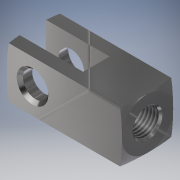
# Autodesk Inventor part: D-14053
Saved by Autodesk Inventor 2017 (Build 210142000, 142)
## iProperties
Category: PARTsolutions
Company: BIMBA
Created: 2016-10-01
Part Number: D-14053
Catalog Web Link: www.cadenas.de
Description: Piston Rod Clevis for Original Line Cylinders - Body-
Vendor: BIMBA
Document SubType Name: Modeling
Designer: psAdmin
Manufacturer: BIMBA
Mass: 70.1826 g
Surface Area: 47.8008 cm^2
Volume: 8.94045 cm^3
Density: 7.85 g/cm^3
Material: Steel, Galvanized
Appearance: Galvanized
PSOL_IDENT_0: {$CADENAS_DATA\23d-libs\bimba\bimba\bimba_imperial\bimba_full_line\original_line_cylinders\accessori
PSOL_IDENT_1: es\piston_rod_clevis_body.prj},202 {VTYP=3D},{NB=D-14053},{LINA=D-14053},{NN=Piston Rod Clevis for O
PSOL_IDENT_2: riginal Line Cylinders - Body},{DATE=22.09.2016 13:52:23},{GEOMDATE=06.12.2012 07:16:06},{VERSION=},
PSOL_IDENT_3: {LINEID=40},{LINESUBID=-1},{WBVAR=}  {NB=D-14053},{LINA=D-14053},{KT=DUMMY},{PN=D-14053},{L=1.688000
PSOL_IDENT_4: 00},{L1=1.31200000},{L2=0.75000000},{W=0.38750000},{W1=0.75000000},{DIA1=0.37200000},{DIA1CS=0.04500
PSOL_IDENT_5: 000},{DIA2=0.75000000},{DIA3=0.39060000},{CS=90.00000000},{CDP=0.03000000},{AN=30.00000000},{NDM=0.4
PSOL_IDENT_6: 3750000},{CODE=UNF},{NDMDP=0.62000000},{COLOR=0.75,0.75,0.75,0.00}
NN: Piston Rod Clevis for Original Line Cylinders - Body
NB: D-14053
NBSYN: $PN.
LINA: D-14053
PN: D-14053
L: 1.68800000
L1: 1.31200000
L2: 0.75000000
W: 0.38750000
W1: 0.75000000
DIA1: 0.37200000
DIA1CS: 0.04500000
DIA2: 0.75000000
DIA3: 0.39060000
CS: 90.00000000
CDP: 0.03000000
AN: 30.00000000
NDM: 0.43750000
CODE: UNF
NDMDP: 0.62000000
SUPPLIER: BIMBA
ARTICLENO: D-14053
BOMINFO: D-14053
CREATOR: CADENAS GmbH
Title: D-14053
Author: Cadenas PARTsolutions
Autodesk Inventor part; units mm, degrees
sketch "Sketch_1" plane through (0, 0, 0) normal (0, 0, 1) x (1, 0, 0)
  line L0 (-9.5504, -9.525) -> (33.3248, -9.525)
  line L1 (33.3248, -9.525) -> (33.3248, 9.525)
  line L2 (33.3248, 9.525) -> (-9.5504, 9.525)
  line L3 (-9.5504, 9.525) -> (-9.5504, -9.525)
  constraints: 8 end point
extrude "Extrusion1" add sketch "Sketch_1" along normal mid plane 19.05
sketch "Sketch_2" plane through (0, 0, 0) normal (0, 1, 0) x (-1, 0, 0)
  line L0 (9.5504, 4.9212) -> (-14.2748, 4.9212)
  line L1 (-14.2748, 4.9212) -> (-14.2748, -4.9212)
  line L2 (-14.2748, -4.9212) -> (9.5504, -4.9212)
  line L3 (9.5504, -4.9212) -> (9.5504, 4.9212)
  constraints: 8 end point
extrude "Extrusion2" cut sketch "Sketch_2" along normal mid plane 19.05
sketch "Sketch_3" plane through (0, 0, 0) normal (0, 0, 1) x (1, 0, 0)
  line L0 (33.3248, 0) -> (17.5768, 0)
  line L1 (17.5768, 0) -> (17.5768, 4.8692)
  line L2 (17.5768, 4.8692) -> (32.6377, 4.8692)
  line L3 (32.6377, 4.8692) -> (33.3248, 5.5563)
  line L4 (33.3248, 5.5563) -> (33.3248, 0)
  line L5 (33.3248, 0) -> (17.5768, 0)
  constraints: 12 end point
revolve "Revolution1" cut sketch "Sketch_3" angle 360 about axis through (33.3248, 0, 0) along (1, 0, 0)
thread "Thread1" size "7/16-20 UNF" class "2B" standard "ANSI Unified Screw Threads" full length
sketch "Sketch5" plane through (17.5768, 0, 0) normal (1, 0, 0) x (0, 0, -1)
  point P0 (0, 0)
hole "Hole1" at (17.5768, 0, 0) direction (-1, 0, 0) diameter 9.9212 depth 3.302
sketch "Sketch_5" plane through (0, 0, 0) normal (1, 0, 0) x (0, 1, 0)
  line L0 (0, -9.525) -> (0, 9.525)
  line L1 (0, 9.525) -> (5.8674, 9.525)
  line L2 (5.8674, 9.525) -> (4.7244, 8.382)
  line L3 (4.7244, 8.382) -> (4.7244, -8.382)
  line L4 (4.7244, -8.382) -> (5.8674, -9.525)
  line L5 (5.8674, -9.525) -> (0, -9.525)
  line L6 (0, -9.525) -> (0, 9.525)
  constraints: 14 end point
revolve "Revolution2" cut sketch "Sketch_5" angle 360 about axis through (0, 0, -9.525) along (0, 0, -1)
sketch "Sketch_9" plane through (0, 0, 0) normal (0, 0, 1) x (1, 0, 0)
  line L0 (42.8498, 0) -> (33.3248, 0)
  line L1 (33.3248, 0) -> (33.3248, 9.525)
  arc A0 (33.3248, 9.525) -> (30.7848, 19.05) centre (-3.664, 4.7625) ccw
  line L2 (30.7848, 19.05) -> (42.8498, 19.05)
  line L3 (42.8498, 19.05) -> (42.8498, 0)
  line L4 (42.8498, 0) -> (33.3248, 0)
  constraints: 10 end point, 2 point on circle, 1 centre point
revolve "Revolution3" cut sketch "Sketch_9" angle 360 about axis through (42.8498, 0, 0) along (1, 0, 0)
sketch "Sketch_10" plane through (0, 0, 0) normal (0, 0, 1) x (1, 0, 0)
  line L0 (-9.5504, 0) -> (-19.0754, 0)
  line L1 (-19.0754, 0) -> (-19.0754, 19.05)
  line L2 (-19.0754, 19.05) -> (-7.0104, 19.05)
  arc A0 (-7.0104, 19.05) -> (-9.5504, 9.525) centre (27.4383, 4.7625) ccw
  line L3 (-9.5504, 9.525) -> (-9.5504, 0)
  line L4 (-9.5504, 0) -> (-19.0754, 0)
  constraints: 10 end point, 2 point on circle, 1 centre point
revolve "Revolution4" cut sketch "Sketch_10" angle 360 about axis through (-9.5504, 0, 0) along (1, 0, 0)
ref_plane "dummy_XY" through (0, 0, 0) normal (0, 0, 1) x (1, 0, 0)
ref_plane "dummy_YZ" through (0, 0, 0) normal (1, 0, 0) x (0, 1, 0)
ref_plane "dummy_ZX" through (0, 0, 0) normal (0, 1, 0) x (0, 0, 1)
ref_plane "h1_XY" through (-9.5504, 9.525, 0) normal (0, 0, 1) x (1, 0, 0)
ref_plane "h1_YZ" through (-9.5504, 9.525, 0) normal (1, 0, 0) x (0, 1, 0)
ref_plane "h1_ZX" through (-9.5504, 9.525, 0) normal (0, 1, 0) x (0, 0, 1)
ref_plane "h2_XY" through (-9.5504, -9.525, 0) normal (0, 0, 1) x (1, 0, 0)
ref_plane "h2_YZ" through (-9.5504, -9.525, 0) normal (1, 0, 0) x (0, 1, 0)
ref_plane "h2_ZX" through (-9.5504, -9.525, 0) normal (0, 1, 0) x (0, 0, 1)
ref_plane "l1_XY" through (33.3248, 9.525, 0) normal (0, 0, 1) x (1, 0, 0)
ref_plane "l1_YZ" through (33.3248, 9.525, 0) normal (1, 0, 0) x (0, 1, 0)
ref_plane "l1_ZX" through (33.3248, 9.525, 0) normal (0, 1, 0) x (0, 0, 1)
ref_plane "l11_XY" through (33.3248, 9.525, 0) normal (0, 0, 1) x (1, 0, 0)
ref_plane "l11_YZ" through (33.3248, 9.525, 0) normal (1, 0, 0) x (0, 1, 0)
ref_plane "l11_ZX" through (33.3248, 9.525, 0) normal (0, 1, 0) x (0, 0, 1)
ref_plane "l12_XY" through (0, 9.525, 0) normal (0, 0, 1) x (1, 0, 0)
ref_plane "l12_YZ" through (0, 9.525, 0) normal (1, 0, 0) x (0, 1, 0)
ref_plane "l12_ZX" through (0, 9.525, 0) normal (0, 1, 0) x (0, 0, 1)
ref_plane "l2_XY" through (-9.5504, 9.525, 0) normal (0, 0, 1) x (1, 0, 0)
ref_plane "l2_YZ" through (-9.5504, 9.525, 0) normal (1, 0, 0) x (0, 1, 0)
ref_plane "l2_ZX" through (-9.5504, 9.525, 0) normal (0, 1, 0) x (0, 0, 1)
ref_plane "l21_XY" through (33.3248, 0, 0) normal (0, 1, 0) x (1, 0, 0)
ref_plane "l21_YZ" through (33.3248, 0, 0) normal (1, 0, 0) x (0, 0, -1)
ref_plane "l21_ZX" through (33.3248, 0, 0) normal (0, 0, -1) x (0, 1, 0)
ref_plane "l22_XY" through (14.2748, 0, 0) normal (0, 1, 0) x (1, 0, 0)
ref_plane "l22_YZ" through (14.2748, 0, 0) normal (1, 0, 0) x (0, 0, -1)
ref_plane "l22_ZX" through (14.2748, 0, 0) normal (0, 0, -1) x (0, 1, 0)
ref_plane "piston_rod_clevis_XY" through (33.3248, 0, 0) normal (1, 0, 0) x (0, 0, -1)
ref_plane "piston_rod_clevis_YZ" through (33.3248, 0, 0) normal (0, 0, -1) x (0, 1, 0)
ref_plane "piston_rod_clevis_ZX" through (33.3248, 0, 0) normal (0, 1, 0) x (1, 0, 0)
ref_plane "rod_clevis_body_XY" through (0, 0, 0) normal (0, 0, 1) x (1, 0, 0)
ref_plane "rod_clevis_body_YZ" through (0, 0, 0) normal (1, 0, 0) x (0, 1, 0)
ref_plane "rod_clevis_body_ZX" through (0, 0, 0) normal (0, 1, 0) x (0, 0, 1)
ref_plane "th1_XY" through (33.3248, 5.5563, 0) normal (0, 0, 1) x (1, 0, 0)
ref_plane "th1_YZ" through (33.3248, 5.5563, 0) normal (1, 0, 0) x (0, 1, 0)
ref_plane "th1_ZX" through (33.3248, 5.5563, 0) normal (0, 1, 0) x (0, 0, 1)
ref_plane "th2_XY" through (33.3248, -5.5563, 0) normal (0, 0, 1) x (1, 0, 0)
ref_plane "th2_YZ" through (33.3248, -5.5563, 0) normal (1, 0, 0) x (0, 1, 0)
ref_plane "th2_ZX" through (33.3248, -5.5563, 0) normal (0, 1, 0) x (0, 0, 1)
ref_plane "to_cylinder_XY" through (14.2748, 0, 0) normal (1, 0, 0) x (0, 0, -1)
ref_plane "to_cylinder_YZ" through (14.2748, 0, 0) normal (0, 0, -1) x (0, 1, 0)
ref_plane "to_cylinder_ZX" through (14.2748, 0, 0) normal (0, 1, 0) x (1, 0, 0)
ref_plane "w1_XY" through (33.3248, 0, -9.525) normal (0, 1, 0) x (1, 0, 0)
ref_plane "w1_YZ" through (33.3248, 0, -9.525) normal (1, 0, 0) x (0, 0, -1)
ref_plane "w1_ZX" through (33.3248, 0, -9.525) normal (0, 0, -1) x (0, 1, 0)
ref_plane "w11_XY" through (-9.5504, 0, -4.9212) normal (0, 1, 0) x (1, 0, 0)
ref_plane "w11_YZ" through (-9.5504, 0, -4.9212) normal (1, 0, 0) x (0, 0, -1)
ref_plane "w11_ZX" through (-9.5504, 0, -4.9212) normal (0, 0, -1) x (0, 1, 0)
ref_plane "w12_XY" through (-9.5504, 0, 4.9212) normal (0, 1, 0) x (1, 0, 0)
ref_plane "w12_YZ" through (-9.5504, 0, 4.9212) normal (1, 0, 0) x (0, 0, -1)
ref_plane "w12_ZX" through (-9.5504, 0, 4.9212) normal (0, 0, -1) x (0, 1, 0)
ref_plane "w2_XY" through (33.3248, 0, 9.525) normal (0, 1, 0) x (1, 0, 0)
ref_plane "w2_YZ" through (33.3248, 0, 9.525) normal (1, 0, 0) x (0, 0, -1)
ref_plane "w2_ZX" through (33.3248, 0, 9.525) normal (0, 0, -1) x (0, 1, 0)
body "Solid1"
